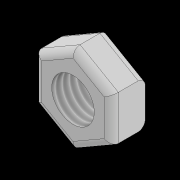
# Autodesk Inventor part: HexNut_Template
Saved by Autodesk Inventor 2022.2 (Build 262287010, 287A)
## iProperties
Created: 2022-05-24
Part Number: HexNut_Template
Material: Generic
Document SubType Name: Modeling
Designer: Árni Þór Þorgeirsson
Density: 1 g/cm^3
Appearance: Default
Author: Árni Þór Þorgeirsson
Autodesk Inventor part; units mm, degrees
ref_plane "YZ Plane" through (0, 0, 0) normal (1, 0, 0) x (0, 1, 0)
ref_plane "XZ Plane" through (0, 0, 0) normal (0, 1, 0) x (-1, 0, 0)
ref_plane "XY Plane" through (0, 0, 0) normal (0, 0, 1) x (1, 0, 0)
sketch "Sketch1" plane through (0, 0, 0) normal (0, 0, 1) x (1, 0, 0)
  line L0 (2.7, -1.5588) -> (0, -3.1177)
  line L1 (0, -3.1177) -> (-2.7, -1.5588)
  line L2 (-2.7, -1.5588) -> (-2.7, 1.5588)
  line L3 (-2.7, 1.5588) -> (0, 3.1177)
  line L4 (0, 3.1177) -> (2.7, 1.5588)
  line L5 (2.7, 1.5588) -> (2.7, -1.5588)
  circle A0 centre (0, 0) radius 1.5
  dimension "d0" = 5.4
  dimension "d1" = 1.5
  constraints: 12 end point, 2 coincident, 1 centre point, 13 other
  measures "d0" distance between parallel lines of L5 L2
  measures "d1" radius of A0
extrude "Extrusion1" add sketch "Sketch1" along normal blind 2.4
thread "Thread1" size "M3x0.5" class "6H" standard "ISO Metric profile" full length
fillet "Fillet1" radius 0.5 11 edges at (1.35, 2.3383, 2.4) (-1.35, 2.3383, 2.4) (-2.7, 0, 2.4) (-1.35, -2.3383, 2.4) (1.35, -2.3383, 2.4) (2.7, 0, 2.4) (1.35, 2.3383, 0) (-1.35, 2.3383, 0) (-2.7, 0, 0) (-1.35, -2.3383, 0) (1.35, -2.3383, 0)
equation "\"d0\" = Machine_Screw_HexNut_Width"
equation "\"d2\" = Machine_Screw_HexNut_Thickness"
equation "\"Machine_Screw_HexNut_Width\" = 5.4"
equation "\"Machine_Screw_HexNut_Thickness\" = 2.4"
body "Solid1"
